Autodesk Fusion 360 part; units mm, degrees
(part 3 of 3)
sketch "Sketch8" plane through (0, 0, 4) normal (0, 0, 1) x (-1, 0, 0)
  arc A0 (-3.5192, 24.2905) -> (-4.2905, 23.5192) centre (0, 20) ccw
  arc A1 (-4.9606, 23.4245) -> (-4.2905, 23.5192) centre (-4.6771, 23.8363) ccw
  line L0 (-4.9606, 23.4245) -> (-6.1877, 24.2692)
  spline S0 degree 5 poles (-6.1877, 24.2692) (-6.1938, 24.2734) (-6.2062, 24.2817) (-6.2253, 24.2932) (-6.2514, 24.3073) (-6.2853, 24.3231) (-6.3199, 24.3375) (-6.355, 24.3512) (-6.3904, 24.3643) (-6.426, 24.3772) (-6.4618, 24.3897) (-6.4979, 24.4018) (-6.5343, 24.4132) (-6.571, 24.424) (-6.6082, 24.434) (-6.6457, 24.4434) (-6.6834, 24.4523) (-6.7214, 24.4607) (-6.7596, 24.4687) (-6.798, 24.4763) (-6.8365, 24.4835) (-6.8753, 24.4902) (-6.9143, 24.4965) (-6.9535, 24.5023) (-6.9928, 24.5077) (-7.0324, 24.5126) (-7.0722, 24.5171) (-7.1121, 24.5212) (-7.1522, 24.5249) (-7.1924, 24.5282) (-7.2328, 24.5311) (-7.2733, 24.5336) (-7.314, 24.5357) (-7.3548, 24.5374) (-7.3957, 24.5387) (-7.4368, 24.5396) (-7.478, 24.5402) (-7.5194, 24.5403) (-7.5608, 24.5401) (-7.6024, 24.5395) (-7.6441, 24.5386) (-7.6858, 24.5373) (-7.7277, 24.5356) (-7.7697, 24.5335) (-7.8118, 24.5311) (-7.854, 24.5283) (-7.8963, 24.5252) (-7.9386, 24.5217) (-7.9811, 24.5178) (-8.0236, 24.5136) (-8.0662, 24.509) (-8.1089, 24.5041) (-8.1517, 24.4988) (-8.1945, 24.4932) (-8.2374, 24.4872) (-8.2804, 24.4809) (-8.3234, 24.4742) (-8.3665, 24.4672) (-8.4097, 24.4598) (-8.4529, 24.4521) (-8.4961, 24.444) (-8.5394, 24.4357) (-8.5828, 24.4269) (-8.6261, 24.4179) (-8.6696, 24.4084) (-8.7131, 24.3987) (-8.7566, 24.3886) (-8.8001, 24.3782) (-8.8437, 24.3675) (-8.8873, 24.3564) (-8.9309, 24.345) (-8.9658, 24.3356) (-8.992, 24.3284) (-9.0095, 24.3235) (-9.0182, 24.321) knots 0 0 0 0 0 0 0.01428571 0.02857143 0.04285714 0.05714286 0.07142857 0.08571429 0.1 0.11428571 0.12857143 0.14285714 0.15714286 0.17142857 0.18571429 0.2 0.21428571 0.22857143 0.24285714 0.25714286 0.27142857 0.28571429 0.3 0.31428571 0.32857143 0.34285714 0.35714286 0.37142857 0.38571429 0.4 0.41428571 0.42857143 0.44285714 0.45714286 0.47142857 0.48571429 0.5 0.51428571 0.52857143 0.54285714 0.55714286 0.57142857 0.58571429 0.6 0.61428571 0.62857143 0.64285714 0.65714286 0.67142857 0.68571429 0.7 0.71428571 0.72857143 0.74285714 0.75714286 0.77142857 0.78571429 0.8 0.81428571 0.82857143 0.84285714 0.85714286 0.87142857 0.88571429 0.9 0.91428571 0.92857143 0.94285714 0.95714286 0.97142857 0.98571429 1 1 1 1 1 1
  arc A2 (-9.0182, 24.321) -> (-9.4323, 23.3214) centre (0, 20) ccw
  spline S1 degree 5 poles (-9.4323, 23.3214) (-9.4278, 23.3135) (-9.4189, 23.2977) (-9.4055, 23.2741) (-9.3874, 23.2427) (-9.3647, 23.2038) (-9.3417, 23.1652) (-9.3185, 23.1268) (-9.295, 23.0886) (-9.2714, 23.0507) (-9.2476, 23.0131) (-9.2235, 22.9757) (-9.1992, 22.9386) (-9.1748, 22.9018) (-9.1501, 22.8652) (-9.1252, 22.829) (-9.1001, 22.793) (-9.0748, 22.7573) (-9.0493, 22.7218) (-9.0236, 22.6867) (-8.9977, 22.6518) (-8.9716, 22.6173) (-8.9453, 22.583) (-8.9187, 22.549) (-8.892, 22.5153) (-8.8651, 22.482) (-8.8381, 22.4489) (-8.8108, 22.4162) (-8.7833, 22.3837) (-8.7556, 22.3516) (-8.7278, 22.3198) (-8.6997, 22.2883) (-8.6715, 22.2572) (-8.643, 22.2264) (-8.6144, 22.1959) (-8.5856, 22.1658) (-8.5567, 22.1359) (-8.5275, 22.1065) (-8.4981, 22.0774) (-8.4686, 22.0486) (-8.4389, 22.0202) (-8.409, 21.9922) (-8.379, 21.9646) (-8.3487, 21.9373) (-8.3183, 21.9104) (-8.2877, 21.8839) (-8.2569, 21.8578) (-8.226, 21.8321) (-8.1948, 21.8067) (-8.1636, 21.7818) (-8.1321, 21.7573) (-8.1005, 21.7332) (-8.0686, 21.7096) (-8.0366, 21.6865) (-8.0045, 21.6639) (-7.9721, 21.6417) (-7.9396, 21.6199) (-7.907, 21.5985) (-7.8742, 21.5776) (-7.8412, 21.5572) (-7.808, 21.5374) (-7.7746, 21.5182) (-7.741, 21.4998) (-7.7072, 21.4822) (-7.6732, 21.4652) (-7.639, 21.4487) (-7.6047, 21.4326) (-7.5704, 21.4169) (-7.5359, 21.4017) (-7.5013, 21.3875) (-7.4662, 21.3747) (-7.4377, 21.3661) (-7.416, 21.3609) (-7.4015, 21.3579) (-7.3941, 21.3565) knots -1 -1 -1 -1 -1 -1 -0.98571429 -0.97142857 -0.95714286 -0.94285714 -0.92857143 -0.91428571 -0.9 -0.88571429 -0.87142857 -0.85714286 -0.84285714 -0.82857143 -0.81428571 -0.8 -0.78571429 -0.77142857 -0.75714286 -0.74285714 -0.72857143 -0.71428571 -0.7 -0.68571429 -0.67142857 -0.65714286 -0.64285714 -0.62857143 -0.61428571 -0.6 -0.58571429 -0.57142857 -0.55714286 -0.54285714 -0.52857143 -0.51428571 -0.5 -0.48571429 -0.47142857 -0.45714286 -0.44285714 -0.42857143 -0.41428571 -0.4 -0.38571429 -0.37142857 -0.35714286 -0.34285714 -0.32857143 -0.31428571 -0.3 -0.28571429 -0.27142857 -0.25714286 -0.24285714 -0.22857143 -0.21428571 -0.2 -0.18571429 -0.17142857 -0.15714286 -0.14285714 -0.12857143 -0.11428571 -0.1 -0.08571429 -0.07142857 -0.05714286 -0.04285714 -0.02857143 -0.01428571 0 0 0 0 0 0
  line L1 (-7.3941, 21.3565) -> (-5.9292, 21.0862)
  arc A3 (-5.5223, 20.5454) -> (-5.9292, 21.0862) centre (-6.0199, 20.5945) ccw
  arc A4 (-5.5223, 20.5454) -> (-5.5223, 19.4546) centre (0, 20) ccw
  arc A5 (-5.9292, 18.9138) -> (-5.5223, 19.4546) centre (-6.0199, 19.4055) ccw
  line L2 (-5.9292, 18.9138) -> (-7.3941, 18.6435)
  spline S2 degree 5 poles (-7.3941, 18.6435) (-7.4015, 18.6421) (-7.416, 18.6391) (-7.4377, 18.6339) (-7.4662, 18.6253) (-7.5013, 18.6125) (-7.5359, 18.5983) (-7.5704, 18.5831) (-7.6047, 18.5674) (-7.639, 18.5513) (-7.6732, 18.5348) (-7.7072, 18.5178) (-7.741, 18.5002) (-7.7746, 18.4818) (-7.808, 18.4626) (-7.8412, 18.4428) (-7.8742, 18.4224) (-7.907, 18.4015) (-7.9396, 18.3801) (-7.9721, 18.3583) (-8.0045, 18.3361) (-8.0366, 18.3135) (-8.0686, 18.2904) (-8.1005, 18.2668) (-8.1321, 18.2427) (-8.1636, 18.2182) (-8.1948, 18.1933) (-8.226, 18.1679) (-8.2569, 18.1422) (-8.2877, 18.1161) (-8.3183, 18.0896) (-8.3487, 18.0627) (-8.379, 18.0354) (-8.409, 18.0078) (-8.4389, 17.9798) (-8.4686, 17.9514) (-8.4981, 17.9226) (-8.5275, 17.8935) (-8.5567, 17.8641) (-8.5856, 17.8343) (-8.6144, 17.8041) (-8.643, 17.7736) (-8.6715, 17.7428) (-8.6997, 17.7117) (-8.7278, 17.6802) (-8.7556, 17.6484) (-8.7833, 17.6163) (-8.8108, 17.5838) (-8.8381, 17.5511) (-8.8651, 17.518) (-8.892, 17.4847) (-8.9187, 17.451) (-8.9453, 17.417) (-8.9716, 17.3827) (-8.9977, 17.3482) (-9.0236, 17.3133) (-9.0493, 17.2782) (-9.0748, 17.2427) (-9.1001, 17.207) (-9.1252, 17.171) (-9.1501, 17.1348) (-9.1748, 17.0982) (-9.1992, 17.0614) (-9.2235, 17.0243) (-9.2476, 16.9869) (-9.2714, 16.9493) (-9.295, 16.9114) (-9.3185, 16.8733) (-9.3417, 16.8348) (-9.3647, 16.7962) (-9.3874, 16.7573) (-9.4055, 16.7259) (-9.4189, 16.7023) (-9.4278, 16.6865) (-9.4323, 16.6786) knots 0 0 0 0 0 0 0.01428571 0.02857143 0.04285714 0.05714286 0.07142857 0.08571429 0.1 0.11428571 0.12857143 0.14285714 0.15714286 0.17142857 0.18571429 0.2 0.21428571 0.22857143 0.24285714 0.25714286 0.27142857 0.28571429 0.3 0.31428571 0.32857143 0.34285714 0.35714286 0.37142857 0.38571429 0.4 0.41428571 0.42857143 0.44285714 0.45714286 0.47142857 0.48571429 0.5 0.51428571 0.52857143 0.54285714 0.55714286 0.57142857 0.58571429 0.6 0.61428571 0.62857143 0.64285714 0.65714286 0.67142857 0.68571429 0.7 0.71428571 0.72857143 0.74285714 0.75714286 0.77142857 0.78571429 0.8 0.81428571 0.82857143 0.84285714 0.85714286 0.87142857 0.88571429 0.9 0.91428571 0.92857143 0.94285714 0.95714286 0.97142857 0.98571429 1 1 1 1 1 1
  arc A6 (-9.4323, 16.6786) -> (-9.0182, 15.679) centre (0, 20) ccw
  spline S3 degree 5 poles (-9.0182, 15.679) (-9.0095, 15.6765) (-8.992, 15.6716) (-8.9658, 15.6644) (-8.9309, 15.655) (-8.8873, 15.6436) (-8.8437, 15.6325) (-8.8001, 15.6218) (-8.7566, 15.6114) (-8.7131, 15.6013) (-8.6696, 15.5916) (-8.6261, 15.5821) (-8.5828, 15.5731) (-8.5394, 15.5643) (-8.4961, 15.556) (-8.4529, 15.5479) (-8.4097, 15.5402) (-8.3665, 15.5328) (-8.3234, 15.5258) (-8.2804, 15.5191) (-8.2374, 15.5128) (-8.1945, 15.5068) (-8.1517, 15.5012) (-8.1089, 15.4959) (-8.0662, 15.491) (-8.0236, 15.4864) (-7.9811, 15.4822) (-7.9386, 15.4783) (-7.8963, 15.4748) (-7.854, 15.4717) (-7.8118, 15.4689) (-7.7697, 15.4665) (-7.7277, 15.4644) (-7.6858, 15.4627) (-7.6441, 15.4614) (-7.6024, 15.4605) (-7.5608, 15.4599) (-7.5194, 15.4597) (-7.478, 15.4598) (-7.4368, 15.4604) (-7.3957, 15.4613) (-7.3548, 15.4626) (-7.314, 15.4643) (-7.2733, 15.4664) (-7.2328, 15.4689) (-7.1924, 15.4718) (-7.1522, 15.4751) (-7.1121, 15.4788) (-7.0722, 15.4829) (-7.0324, 15.4874) (-6.9928, 15.4923) (-6.9535, 15.4977) (-6.9143, 15.5035) (-6.8753, 15.5098) (-6.8365, 15.5165) (-6.798, 15.5237) (-6.7596, 15.5313) (-6.7214, 15.5393) (-6.6834, 15.5477) (-6.6457, 15.5566) (-6.6082, 15.566) (-6.571, 15.576) (-6.5343, 15.5868) (-6.4979, 15.5982) (-6.4618, 15.6103) (-6.426, 15.6228) (-6.3904, 15.6357) (-6.355, 15.6488) (-6.3199, 15.6625) (-6.2853, 15.6769) (-6.2514, 15.6927) (-6.2253, 15.7068) (-6.2062, 15.7183) (-6.1938, 15.7266) (-6.1877, 15.7308) knots -1 -1 -1 -1 -1 -1 -0.98571429 -0.97142857 -0.95714286 -0.94285714 -0.92857143 -0.91428571 -0.9 -0.88571429 -0.87142857 -0.85714286 -0.84285714 -0.82857143 -0.81428571 -0.8 -0.78571429 -0.77142857 -0.75714286 -0.74285714 -0.72857143 -0.71428571 -0.7 -0.68571429 -0.67142857 -0.65714286 -0.64285714 -0.62857143 -0.61428571 -0.6 -0.58571429 -0.57142857 -0.55714286 -0.54285714 -0.52857143 -0.51428571 -0.5 -0.48571429 -0.47142857 -0.45714286 -0.44285714 -0.42857143 -0.41428571 -0.4 -0.38571429 -0.37142857 -0.35714286 -0.34285714 -0.32857143 -0.31428571 -0.3 -0.28571429 -0.27142857 -0.25714286 -0.24285714 -0.22857143 -0.21428571 -0.2 -0.18571429 -0.17142857 -0.15714286 -0.14285714 -0.12857143 -0.11428571 -0.1 -0.08571429 -0.07142857 -0.05714286 -0.04285714 -0.02857143 -0.01428571 0 0 0 0 0 0
  line L3 (-6.1877, 15.7308) -> (-4.9606, 16.5755)
  arc A7 (-4.2905, 16.4808) -> (-4.9606, 16.5755) centre (-4.6771, 16.1637) ccw
  arc A8 (-4.2905, 16.4808) -> (-3.5192, 15.7095) centre (0, 20) ccw
  arc A9 (-3.4245, 15.0394) -> (-3.5192, 15.7095) centre (-3.8363, 15.3229) ccw
  line L4 (-3.4245, 15.0394) -> (-4.2692, 13.8123)
  spline S4 degree 5 poles (-4.2692, 13.8123) (-4.2734, 13.8062) (-4.2817, 13.7938) (-4.2932, 13.7747) (-4.3073, 13.7486) (-4.3231, 13.7147) (-4.3375, 13.6801) (-4.3512, 13.645) (-4.3643, 13.6096) (-4.3772, 13.574) (-4.3897, 13.5382) (-4.4018, 13.5021) (-4.4132, 13.4657) (-4.424, 13.429) (-4.434, 13.3918) (-4.4434, 13.3543) (-4.4523, 13.3166) (-4.4607, 13.2786) (-4.4687, 13.2404) (-4.4763, 13.202) (-4.4835, 13.1635) (-4.4902, 13.1247) (-4.4965, 13.0857) (-4.5023, 13.0465) (-4.5077, 13.0072) (-4.5126, 12.9676) (-4.5171, 12.9278) (-4.5212, 12.8879) (-4.5249, 12.8478) (-4.5282, 12.8076) (-4.5311, 12.7672) (-4.5336, 12.7267) (-4.5357, 12.686) (-4.5374, 12.6452) (-4.5387, 12.6043) (-4.5396, 12.5632) (-4.5402, 12.522) (-4.5403, 12.4806) (-4.5401, 12.4392) (-4.5395, 12.3976) (-4.5386, 12.3559) (-4.5373, 12.3142) (-4.5356, 12.2723) (-4.5335, 12.2303) (-4.5311, 12.1882) (-4.5283, 12.146) (-4.5252, 12.1037) (-4.5217, 12.0614) (-4.5178, 12.0189) (-4.5136, 11.9764) (-4.509, 11.9338) (-4.5041, 11.8911) (-4.4988, 11.8483) (-4.4932, 11.8055) (-4.4872, 11.7626) (-4.4809, 11.7196) (-4.4742, 11.6766) (-4.4672, 11.6335) (-4.4598, 11.5903) (-4.4521, 11.5471) (-4.444, 11.5039) (-4.4357, 11.4606) (-4.4269, 11.4172) (-4.4179, 11.3739) (-4.4084, 11.3304) (-4.3987, 11.2869) (-4.3886, 11.2434) (-4.3782, 11.1999) (-4.3675, 11.1563) (-4.3564, 11.1127) (-4.345, 11.0691) (-4.3356, 11.0342) (-4.3284, 11.008) (-4.3235, 10.9905) (-4.321, 10.9818) knots 0 0 0 0 0 0 0.01428571 0.02857143 0.04285714 0.05714286 0.07142857 0.08571429 0.1 0.11428571 0.12857143 0.14285714 0.15714286 0.17142857 0.18571429 0.2 0.21428571 0.22857143 0.24285714 0.25714286 0.27142857 0.28571429 0.3 0.31428571 0.32857143 0.34285714 0.35714286 0.37142857 0.38571429 0.4 0.41428571 0.42857143 0.44285714 0.45714286 0.47142857 0.48571429 0.5 0.51428571 0.52857143 0.54285714 0.55714286 0.57142857 0.58571429 0.6 0.61428571 0.62857143 0.64285714 0.65714286 0.67142857 0.68571429 0.7 0.71428571 0.72857143 0.74285714 0.75714286 0.77142857 0.78571429 0.8 0.81428571 0.82857143 0.84285714 0.85714286 0.87142857 0.88571429 0.9 0.91428571 0.92857143 0.94285714 0.95714286 0.97142857 0.98571429 1 1 1 1 1 1
  arc A10 (-4.321, 10.9818) -> (-3.3214, 10.5677) centre (0, 20) ccw
  spline S5 degree 5 poles (-3.3214, 10.5677) (-3.3135, 10.5722) (-3.2977, 10.5811) (-3.2741, 10.5945) (-3.2427, 10.6126) (-3.2038, 10.6353) (-3.1652, 10.6583) (-3.1267, 10.6815) (-3.0886, 10.705) (-3.0507, 10.7286) (-3.0131, 10.7524) (-2.9757, 10.7765) (-2.9386, 10.8008) (-2.9018, 10.8252) (-2.8652, 10.8499) (-2.829, 10.8748) (-2.793, 10.8999) (-2.7573, 10.9252) (-2.7218, 10.9507) (-2.6867, 10.9764) (-2.6518, 11.0023) (-2.6173, 11.0284) (-2.583, 11.0547) (-2.549, 11.0813) (-2.5153, 11.108) (-2.482, 11.1349) (-2.4489, 11.1619) (-2.4162, 11.1892) (-2.3837, 11.2167) (-2.3516, 11.2444) (-2.3198, 11.2722) (-2.2883, 11.3003) (-2.2572, 11.3285) (-2.2264, 11.357) (-2.1959, 11.3856) (-2.1657, 11.4144) (-2.1359, 11.4433) (-2.1065, 11.4725) (-2.0774, 11.5019) (-2.0486, 11.5314) (-2.0202, 11.5611) (-1.9922, 11.591) (-1.9646, 11.621) (-1.9373, 11.6513) (-1.9104, 11.6817) (-1.8839, 11.7123) (-1.8578, 11.7431) (-1.8321, 11.774) (-1.8067, 11.8052) (-1.7818, 11.8364) (-1.7573, 11.8679) (-1.7332, 11.8995) (-1.7096, 11.9314) (-1.6865, 11.9634) (-1.6639, 11.9955) (-1.6417, 12.0279) (-1.6199, 12.0604) (-1.5985, 12.093) (-1.5776, 12.1258) (-1.5572, 12.1588) (-1.5374, 12.192) (-1.5182, 12.2254) (-1.4998, 12.259) (-1.4822, 12.2928) (-1.4652, 12.3268) (-1.4487, 12.361) (-1.4326, 12.3953) (-1.4169, 12.4296) (-1.4017, 12.4641) (-1.3875, 12.4987) (-1.3747, 12.5338) (-1.3661, 12.5623) (-1.3609, 12.584) (-1.3579, 12.5985) (-1.3565, 12.6059) knots -1 -1 -1 -1 -1 -1 -0.98571429 -0.97142857 -0.95714286 -0.94285714 -0.92857143 -0.91428571 -0.9 -0.88571429 -0.87142857 -0.85714286 -0.84285714 -0.82857143 -0.81428571 -0.8 -0.78571429 -0.77142857 -0.75714286 -0.74285714 -0.72857143 -0.71428571 -0.7 -0.68571429 -0.67142857 -0.65714286 -0.64285714 -0.62857143 -0.61428571 -0.6 -0.58571429 -0.57142857 -0.55714286 -0.54285714 -0.52857143 -0.51428571 -0.5 -0.48571429 -0.47142857 -0.45714286 -0.44285714 -0.42857143 -0.41428571 -0.4 -0.38571429 -0.37142857 -0.35714286 -0.34285714 -0.32857143 -0.31428571 -0.3 -0.28571429 -0.27142857 -0.25714286 -0.24285714 -0.22857143 -0.21428571 -0.2 -0.18571429 -0.17142857 -0.15714286 -0.14285714 -0.12857143 -0.11428571 -0.1 -0.08571429 -0.07142857 -0.05714286 -0.04285714 -0.02857143 -0.01428571 0 0 0 0 0 0
  line L5 (-1.3565, 12.6059) -> (-1.0862, 14.0708)
  arc A11 (-0.5454, 14.4777) -> (-1.0862, 14.0708) centre (-0.5945, 13.9801) ccw
  arc A12 (-0.5454, 14.4777) -> (0.5454, 14.4777) centre (0, 20) ccw
  arc A13 (1.0862, 14.0708) -> (0.5454, 14.4777) centre (0.5945, 13.9801) ccw
  line L6 (1.0862, 14.0708) -> (1.3565, 12.6059)
  spline S6 degree 5 poles (1.3565, 12.6059) (1.3579, 12.5985) (1.3609, 12.584) (1.3661, 12.5623) (1.3747, 12.5338) (1.3875, 12.4987) (1.4017, 12.4641) (1.4169, 12.4296) (1.4326, 12.3953) (1.4487, 12.361) (1.4652, 12.3268) (1.4822, 12.2928) (1.4998, 12.259) (1.5182, 12.2254) (1.5374, 12.192) (1.5572, 12.1588) (1.5776, 12.1258) (1.5985, 12.093) (1.6199, 12.0604) (1.6417, 12.0279) (1.6639, 11.9955) (1.6865, 11.9634) (1.7096, 11.9314) (1.7332, 11.8995) (1.7573, 11.8679) (1.7818, 11.8364) (1.8067, 11.8052) (1.8321, 11.774) (1.8578, 11.7431) (1.8839, 11.7123) (1.9104, 11.6817) (1.9373, 11.6513) (1.9646, 11.621) (1.9922, 11.591) (2.0202, 11.5611) (2.0486, 11.5314) (2.0774, 11.5019) (2.1065, 11.4725) (2.1359, 11.4433) (2.1657, 11.4144) (2.1959, 11.3856) (2.2264, 11.357) (2.2572, 11.3285) (2.2883, 11.3003) (2.3198, 11.2722) (2.3516, 11.2444) (2.3837, 11.2167) (2.4162, 11.1892) (2.4489, 11.1619) (2.482, 11.1349) (2.5153, 11.108) (2.549, 11.0813) (2.583, 11.0547) (2.6173, 11.0284) (2.6518, 11.0023) (2.6867, 10.9764) (2.7218, 10.9507) (2.7573, 10.9252) (2.793, 10.8999) (2.829, 10.8748) (2.8652, 10.8499) (2.9018, 10.8252) (2.9386, 10.8008) (2.9757, 10.7765) (3.0131, 10.7524) (3.0507, 10.7286) (3.0886, 10.705) (3.1267, 10.6815) (3.1652, 10.6583) (3.2038, 10.6353) (3.2427, 10.6126) (3.2741, 10.5945) (3.2977, 10.5811) (3.3135, 10.5722) (3.3214, 10.5677) knots 0 0 0 0 0 0 0.01428571 0.02857143 0.04285714 0.05714286 0.07142857 0.08571429 0.1 0.11428571 0.12857143 0.14285714 0.15714286 0.17142857 0.18571429 0.2 0.21428571 0.22857143 0.24285714 0.25714286 0.27142857 0.28571429 0.3 0.31428571 0.32857143 0.34285714 0.35714286 0.37142857 0.38571429 0.4 0.41428571 0.42857143 0.44285714 0.45714286 0.47142857 0.48571429 0.5 0.51428571 0.52857143 0.54285714 0.55714286 0.57142857 0.58571429 0.6 0.61428571 0.62857143 0.64285714 0.65714286 0.67142857 0.68571429 0.7 0.71428571 0.72857143 0.74285714 0.75714286 0.77142857 0.78571429 0.8 0.81428571 0.82857143 0.84285714 0.85714286 0.87142857 0.88571429 0.9 0.91428571 0.92857143 0.94285714 0.95714286 0.97142857 0.98571429 1 1 1 1 1 1
  arc A14 (3.3214, 10.5677) -> (4.321, 10.9818) centre (0, 20) ccw
  spline S7 degree 5 poles (4.321, 10.9818) (4.3235, 10.9905) (4.3284, 11.008) (4.3356, 11.0342) (4.345, 11.0691) (4.3564, 11.1127) (4.3675, 11.1563) (4.3782, 11.1999) (4.3886, 11.2434) (4.3987, 11.2869) (4.4084, 11.3304) (4.4179, 11.3739) (4.4269, 11.4172) (4.4357, 11.4606) (4.444, 11.5039) (4.4521, 11.5471) (4.4598, 11.5903) (4.4672, 11.6335) (4.4742, 11.6766) (4.4809, 11.7196) (4.4872, 11.7626) (4.4932, 11.8055) (4.4988, 11.8483) (4.5041, 11.8911) (4.509, 11.9338) (4.5136, 11.9764) (4.5178, 12.0189) (4.5217, 12.0614) (4.5252, 12.1037) (4.5283, 12.146) (4.5311, 12.1882) (4.5335, 12.2303) (4.5356, 12.2723) (4.5373, 12.3142) (4.5386, 12.3559) (4.5395, 12.3976) (4.5401, 12.4392) (4.5403, 12.4806) (4.5402, 12.522) (4.5396, 12.5632) (4.5387, 12.6043) (4.5374, 12.6452) (4.5357, 12.686) (4.5336, 12.7267) (4.5311, 12.7672) (4.5282, 12.8076) (4.5249, 12.8478) (4.5212, 12.8879) (4.5171, 12.9278) (4.5126, 12.9676) (4.5077, 13.0072) (4.5023, 13.0465) (4.4965, 13.0857) (4.4902, 13.1247) (4.4835, 13.1635) (4.4763, 13.202) (4.4687, 13.2404) (4.4607, 13.2786) (4.4523, 13.3166) (4.4434, 13.3543) (4.434, 13.3918) (4.424, 13.429) (4.4132, 13.4657) (4.4018, 13.5021) (4.3897, 13.5382) (4.3772, 13.574) (4.3643, 13.6096) (4.3512, 13.645) (4.3375, 13.6801) (4.3231, 13.7147) (4.3073, 13.7486) (4.2932, 13.7747) (4.2817, 13.7938) (4.2734, 13.8062) (4.2692, 13.8123) knots -1 -1 -1 -1 -1 -1 -0.98571429 -0.97142857 -0.95714286 -0.94285714 -0.92857143 -0.91428571 -0.9 -0.88571429 -0.87142857 -0.85714286 -0.84285714 -0.82857143 -0.81428571 -0.8 -0.78571429 -0.77142857 -0.75714286 -0.74285714 -0.72857143 -0.71428571 -0.7 -0.68571429 -0.67142857 -0.65714286 -0.64285714 -0.62857143 -0.61428571 -0.6 -0.58571429 -0.57142857 -0.55714286 -0.54285714 -0.52857143 -0.51428571 -0.5 -0.48571429 -0.47142857 -0.45714286 -0.44285714 -0.42857143 -0.41428571 -0.4 -0.38571429 -0.37142857 -0.35714286 -0.34285714 -0.32857143 -0.31428571 -0.3 -0.28571429 -0.27142857 -0.25714286 -0.24285714 -0.22857143 -0.21428571 -0.2 -0.18571429 -0.17142857 -0.15714286 -0.14285714 -0.12857143 -0.11428571 -0.1 -0.08571429 -0.07142857 -0.05714286 -0.04285714 -0.02857143 -0.01428571 0 0 0 0 0 0
  line L7 (4.2692, 13.8123) -> (3.4245, 15.0394)
  arc A15 (3.5192, 15.7095) -> (3.4245, 15.0394) centre (3.8363, 15.3229) ccw
  arc A16 (3.5192, 15.7095) -> (4.2905, 16.4808) centre (0, 20) ccw
  arc A17 (4.9606, 16.5755) -> (4.2905, 16.4808) centre (4.6771, 16.1637) ccw
  line L8 (4.9606, 16.5755) -> (6.1877, 15.7308)
  spline S8 degree 5 poles (6.1877, 15.7308) (6.1938, 15.7266) (6.2062, 15.7183) (6.2253, 15.7068) (6.2514, 15.6927) (6.2853, 15.6769) (6.3199, 15.6625) (6.355, 15.6488) (6.3904, 15.6357) (6.426, 15.6228) (6.4618, 15.6103) (6.4979, 15.5982) (6.5343, 15.5868) (6.571, 15.576) (6.6082, 15.566) (6.6457, 15.5566) (6.6834, 15.5477) (6.7214, 15.5393) (6.7596, 15.5313) (6.798, 15.5237) (6.8365, 15.5165) (6.8753, 15.5098) (6.9143, 15.5035) (6.9535, 15.4977) (6.9928, 15.4923) (7.0324, 15.4874) (7.0722, 15.4829) (7.1121, 15.4788) (7.1522, 15.4751) (7.1924, 15.4718) (7.2328, 15.4689) (7.2733, 15.4664) (7.314, 15.4643) (7.3548, 15.4626) (7.3957, 15.4613) (7.4368, 15.4604) (7.478, 15.4598) (7.5194, 15.4597) (7.5608, 15.4599) (7.6024, 15.4605) (7.6441, 15.4614) (7.6858, 15.4627) (7.7277, 15.4644) (7.7697, 15.4665) (7.8118, 15.4689) (7.854, 15.4717) (7.8963, 15.4748) (7.9386, 15.4783) (7.9811, 15.4822) (8.0236, 15.4864) (8.0662, 15.491) (8.1089, 15.4959) (8.1517, 15.5012) (8.1945, 15.5068) (8.2374, 15.5128) (8.2804, 15.5191) (8.3234, 15.5258) (8.3665, 15.5328) (8.4097, 15.5402) (8.4529, 15.5479) (8.4961, 15.556) (8.5394, 15.5643) (8.5828, 15.5731) (8.6261, 15.5821) (8.6696, 15.5916) (8.7131, 15.6013) (8.7566, 15.6114) (8.8001, 15.6218) (8.8437, 15.6325) (8.8873, 15.6436) (8.9309, 15.655) (8.9658, 15.6644) (8.992, 15.6716) (9.0095, 15.6765) (9.0182, 15.679) knots 0 0 0 0 0 0 0.01428571 0.02857143 0.04285714 0.05714286 0.07142857 0.08571429 0.1 0.11428571 0.12857143 0.14285714 0.15714286 0.17142857 0.18571429 0.2 0.21428571 0.22857143 0.24285714 0.25714286 0.27142857 0.28571429 0.3 0.31428571 0.32857143 0.34285714 0.35714286 0.37142857 0.38571429 0.4 0.41428571 0.42857143 0.44285714 0.45714286 0.47142857 0.48571429 0.5 0.51428571 0.52857143 0.54285714 0.55714286 0.57142857 0.58571429 0.6 0.61428571 0.62857143 0.64285714 0.65714286 0.67142857 0.68571429 0.7 0.71428571 0.72857143 0.74285714 0.75714286 0.77142857 0.78571429 0.8 0.81428571 0.82857143 0.84285714 0.85714286 0.87142857 0.88571429 0.9 0.91428571 0.92857143 0.94285714 0.95714286 0.97142857 0.98571429 1 1 1 1 1 1
  arc A18 (9.0182, 15.679) -> (9.4323, 16.6786) centre (0, 20) ccw
  spline S9 degree 5 poles (9.4323, 16.6786) (9.4278, 16.6865) (9.4189, 16.7023) (9.4055, 16.7259) (9.3874, 16.7573) (9.3647, 16.7962) (9.3417, 16.8348) (9.3185, 16.8733) (9.295, 16.9114) (9.2714, 16.9493) (9.2476, 16.9869) (9.2235, 17.0243) (9.1992, 17.0614) (9.1748, 17.0982) (9.1501, 17.1348) (9.1252, 17.171) (9.1001, 17.207) (9.0748, 17.2427) (9.0493, 17.2782) (9.0236, 17.3133) (8.9977, 17.3482) (8.9716, 17.3827) (8.9453, 17.417) (8.9187, 17.451) (8.892, 17.4847) (8.8651, 17.518) (8.8381, 17.5511) (8.8108, 17.5838) (8.7833, 17.6163) (8.7556, 17.6484) (8.7278, 17.6802) (8.6997, 17.7117) (8.6715, 17.7428) (8.643, 17.7736) (8.6144, 17.8041) (8.5856, 17.8343) (8.5567, 17.8641) (8.5275, 17.8935) (8.4981, 17.9226) (8.4686, 17.9514) (8.4389, 17.9798) (8.409, 18.0078) (8.379, 18.0354) (8.3487, 18.0627) (8.3183, 18.0896) (8.2877, 18.1161) (8.2569, 18.1422) (8.226, 18.1679) (8.1948, 18.1933) (8.1636, 18.2182) (8.1321, 18.2427) (8.1005, 18.2668) (8.0686, 18.2904) (8.0366, 18.3135) (8.0045, 18.3361) (7.9721, 18.3583) (7.9396, 18.3801) (7.907, 18.4015) (7.8742, 18.4224) (7.8412, 18.4428) (7.808, 18.4626) (7.7746, 18.4818) (7.741, 18.5002) (7.7072, 18.5178) (7.6732, 18.5348) (7.639, 18.5513) (7.6047, 18.5674) (7.5704, 18.5831) (7.5359, 18.5983) (7.5013, 18.6125) (7.4662, 18.6253) (7.4377, 18.6339) (7.416, 18.6391) (7.4015, 18.6421) (7.3941, 18.6435) knots -1 -1 -1 -1 -1 -1 -0.98571429 -0.97142857 -0.95714286 -0.94285714 -0.92857143 -0.91428571 -0.9 -0.88571429 -0.87142857 -0.85714286 -0.84285714 -0.82857143 -0.81428571 -0.8 -0.78571429 -0.77142857 -0.75714286 -0.74285714 -0.72857143 -0.71428571 -0.7 -0.68571429 -0.67142857 -0.65714286 -0.64285714 -0.62857143 -0.61428571 -0.6 -0.58571429 -0.57142857 -0.55714286 -0.54285714 -0.52857143 -0.51428571 -0.5 -0.48571429 -0.47142857 -0.45714286 -0.44285714 -0.42857143 -0.41428571 -0.4 -0.38571429 -0.37142857 -0.35714286 -0.34285714 -0.32857143 -0.31428571 -0.3 -0.28571429 -0.27142857 -0.25714286 -0.24285714 -0.22857143 -0.21428571 -0.2 -0.18571429 -0.17142857 -0.15714286 -0.14285714 -0.12857143 -0.11428571 -0.1 -0.08571429 -0.07142857 -0.05714286 -0.04285714 -0.02857143 -0.01428571 0 0 0 0 0 0
  line L9 (7.3941, 18.6435) -> (5.9292, 18.9138)
  arc A19 (5.5223, 19.4546) -> (5.9292, 18.9138) centre (6.0199, 19.4055) ccw
  arc A20 (5.5223, 19.4546) -> (5.5223, 20.5454) centre (0, 20) ccw
  arc A21 (5.9292, 21.0862) -> (5.5223, 20.5454) centre (6.0199, 20.5945) ccw
  line L10 (5.9292, 21.0862) -> (7.3941, 21.3565)
  spline S10 degree 5 poles (7.3941, 21.3565) (7.4015, 21.3579) (7.416, 21.3609) (7.4377, 21.3661) (7.4662, 21.3747) (7.5013, 21.3875) (7.5359, 21.4017) (7.5704, 21.4169) (7.6047, 21.4326) (7.639, 21.4487) (7.6732, 21.4652) (7.7072, 21.4822) (7.741, 21.4998) (7.7746, 21.5182) (7.808, 21.5374) (7.8412, 21.5572) (7.8742, 21.5776) (7.907, 21.5985) (7.9396, 21.6199) (7.9721, 21.6417) (8.0045, 21.6639) (8.0366, 21.6865) (8.0686, 21.7096) (8.1005, 21.7332) (8.1321, 21.7573) (8.1636, 21.7818) (8.1948, 21.8067) (8.226, 21.8321) (8.2569, 21.8578) (8.2877, 21.8839) (8.3183, 21.9104) (8.3487, 21.9373) (8.379, 21.9646) (8.409, 21.9922) (8.4389, 22.0202) (8.4686, 22.0486) (8.4981, 22.0774) (8.5275, 22.1065) (8.5567, 22.1359) (8.5856, 22.1658) (8.6144, 22.1959) (8.643, 22.2264) (8.6715, 22.2572) (8.6997, 22.2883) (8.7278, 22.3198) (8.7556, 22.3516) (8.7833, 22.3837) (8.8108, 22.4162) (8.8381, 22.4489) (8.8651, 22.482) (8.892, 22.5153) (8.9187, 22.549) (8.9453, 22.583) (8.9716, 22.6173) (8.9977, 22.6518) (9.0236, 22.6867) (9.0493, 22.7218) (9.0748, 22.7573) (9.1001, 22.793) (9.1252, 22.829) (9.1501, 22.8652) (9.1748, 22.9018) (9.1992, 22.9386) (9.2235, 22.9757) (9.2476, 23.0131) (9.2714, 23.0507) (9.295, 23.0886) (9.3185, 23.1268) (9.3417, 23.1652) (9.3647, 23.2038) (9.3874, 23.2427) (9.4055, 23.2741) (9.4189, 23.2977) (9.4278, 23.3135) (9.4323, 23.3214) knots 0 0 0 0 0 0 0.01428571 0.02857143 0.04285714 0.05714286 0.07142857 0.08571429 0.1 0.11428571 0.12857143 0.14285714 0.15714286 0.17142857 0.18571429 0.2 0.21428571 0.22857143 0.24285714 0.25714286 0.27142857 0.28571429 0.3 0.31428571 0.32857143 0.34285714 0.35714286 0.37142857 0.38571429 0.4 0.41428571 0.42857143 0.44285714 0.45714286 0.47142857 0.48571429 0.5 0.51428571 0.52857143 0.54285714 0.55714286 0.57142857 0.58571429 0.6 0.61428571 0.62857143 0.64285714 0.65714286 0.67142857 0.68571429 0.7 0.71428571 0.72857143 0.74285714 0.75714286 0.77142857 0.78571429 0.8 0.81428571 0.82857143 0.84285714 0.85714286 0.87142857 0.88571429 0.9 0.91428571 0.92857143 0.94285714 0.95714286 0.97142857 0.98571429 1 1 1 1 1 1
  arc A22 (9.4323, 23.3214) -> (9.0182, 24.321) centre (0, 20) ccw
  spline S11 degree 5 poles (9.0182, 24.321) (9.0095, 24.3235) (8.992, 24.3284) (8.9658, 24.3356) (8.9309, 24.345) (8.8873, 24.3564) (8.8437, 24.3675) (8.8001, 24.3782) (8.7566, 24.3886) (8.7131, 24.3987) (8.6696, 24.4084) (8.6261, 24.4179) (8.5828, 24.4269) (8.5394, 24.4357) (8.4961, 24.444) (8.4529, 24.4521) (8.4097, 24.4598) (8.3665, 24.4672) (8.3234, 24.4742) (8.2804, 24.4809) (8.2374, 24.4872) (8.1945, 24.4932) (8.1517, 24.4988) (8.1089, 24.5041) (8.0662, 24.509) (8.0236, 24.5136) (7.9811, 24.5178) (7.9386, 24.5217) (7.8963, 24.5252) (7.854, 24.5283) (7.8118, 24.5311) (7.7697, 24.5335) (7.7277, 24.5356) (7.6858, 24.5373) (7.6441, 24.5386) (7.6024, 24.5395) (7.5608, 24.5401) (7.5194, 24.5403) (7.478, 24.5402) (7.4368, 24.5396) (7.3957, 24.5387) (7.3548, 24.5374) (7.314, 24.5357) (7.2733, 24.5336) (7.2328, 24.5311) (7.1924, 24.5282) (7.1522, 24.5249) (7.1121, 24.5212) (7.0722, 24.5171) (7.0324, 24.5126) (6.9928, 24.5077) (6.9535, 24.5023) (6.9143, 24.4965) (6.8753, 24.4902) (6.8365, 24.4835) (6.798, 24.4763) (6.7596, 24.4687) (6.7214, 24.4607) (6.6834, 24.4523) (6.6457, 24.4434) (6.6082, 24.434) (6.571, 24.424) (6.5343, 24.4132) (6.4979, 24.4018) (6.4618, 24.3897) (6.426, 24.3772) (6.3904, 24.3643) (6.355, 24.3512) (6.3199, 24.3375) (6.2853, 24.3231) (6.2514, 24.3073) (6.2253, 24.2932) (6.2062, 24.2817) (6.1938, 24.2734) (6.1877, 24.2692) knots -1 -1 -1 -1 -1 -1 -0.98571429 -0.97142857 -0.95714286 -0.94285714 -0.92857143 -0.91428571 -0.9 -0.88571429 -0.87142857 -0.85714286 -0.84285714 -0.82857143 -0.81428571 -0.8 -0.78571429 -0.77142857 -0.75714286 -0.74285714 -0.72857143 -0.71428571 -0.7 -0.68571429 -0.67142857 -0.65714286 -0.64285714 -0.62857143 -0.61428571 -0.6 -0.58571429 -0.57142857 -0.55714286 -0.54285714 -0.52857143 -0.51428571 -0.5 -0.48571429 -0.47142857 -0.45714286 -0.44285714 -0.42857143 -0.41428571 -0.4 -0.38571429 -0.37142857 -0.35714286 -0.34285714 -0.32857143 -0.31428571 -0.3 -0.28571429 -0.27142857 -0.25714286 -0.24285714 -0.22857143 -0.21428571 -0.2 -0.18571429 -0.17142857 -0.15714286 -0.14285714 -0.12857143 -0.11428571 -0.1 -0.08571429 -0.07142857 -0.05714286 -0.04285714 -0.02857143 -0.01428571 0 0 0 0 0 0
  line L11 (6.1877, 24.2692) -> (4.9606, 23.4245)
  arc A23 (4.2905, 23.5192) -> (4.9606, 23.4245) centre (4.6771, 23.8363) ccw
  arc A24 (4.2905, 23.5192) -> (3.5192, 24.2905) centre (0, 20) ccw
  arc A25 (3.4245, 24.9606) -> (3.5192, 24.2905) centre (3.8363, 24.6771) ccw
  line L12 (3.4245, 24.9606) -> (4.2692, 26.1877)
  spline S12 degree 5 poles (4.2692, 26.1877) (4.2734, 26.1938) (4.2817, 26.2062) (4.2932, 26.2253) (4.3073, 26.2514) (4.3231, 26.2853) (4.3375, 26.3199) (4.3512, 26.355) (4.3643, 26.3904) (4.3772, 26.426) (4.3897, 26.4618) (4.4018, 26.4979) (4.4132, 26.5343) (4.424, 26.5711) (4.434, 26.6082) (4.4434, 26.6457) (4.4523, 26.6834) (4.4607, 26.7214) (4.4687, 26.7596) (4.4763, 26.798) (4.4835, 26.8365) (4.4902, 26.8753) (4.4965, 26.9143) (4.5023, 26.9535) (4.5077, 26.9928) (4.5126, 27.0324) (4.5171, 27.0722) (4.5212, 27.1121) (4.5249, 27.1522) (4.5282, 27.1924) (4.5311, 27.2328) (4.5336, 27.2733) (4.5357, 27.314) (4.5374, 27.3548) (4.5387, 27.3957) (4.5396, 27.4368) (4.5402, 27.478) (4.5403, 27.5194) (4.5401, 27.5608) (4.5395, 27.6024) (4.5386, 27.6441) (4.5373, 27.6858) (4.5356, 27.7277) (4.5335, 27.7697) (4.5311, 27.8118) (4.5283, 27.854) (4.5252, 27.8963) (4.5217, 27.9386) (4.5178, 27.9811) (4.5136, 28.0236) (4.509, 28.0662) (4.5041, 28.1089) (4.4988, 28.1517) (4.4932, 28.1945) (4.4872, 28.2374) (4.4809, 28.2804) (4.4742, 28.3234) (4.4672, 28.3665) (4.4598, 28.4097) (4.4521, 28.4529) (4.444, 28.4961) (4.4357, 28.5394) (4.4269, 28.5828) (4.4179, 28.6261) (4.4084, 28.6696) (4.3987, 28.7131) (4.3886, 28.7566) (4.3782, 28.8001) (4.3675, 28.8437) (4.3564, 28.8873) (4.345, 28.9309) (4.3356, 28.9658) (4.3284, 28.992) (4.3235, 29.0095) (4.321, 29.0182) knots 0 0 0 0 0 0 0.01428571 0.02857143 0.04285714 0.05714286 0.07142857 0.08571429 0.1 0.11428571 0.12857143 0.14285714 0.15714286 0.17142857 0.18571429 0.2 0.21428571 0.22857143 0.24285714 0.25714286 0.27142857 0.28571429 0.3 0.31428571 0.32857143 0.34285714 0.35714286 0.37142857 0.38571429 0.4 0.41428571 0.42857143 0.44285714 0.45714286 0.47142857 0.48571429 0.5 0.51428571 0.52857143 0.54285714 0.55714286 0.57142857 0.58571429 0.6 0.61428571 0.62857143 0.64285714 0.65714286 0.67142857 0.68571429 0.7 0.71428571 0.72857143 0.74285714 0.75714286 0.77142857 0.78571429 0.8 0.81428571 0.82857143 0.84285714 0.85714286 0.87142857 0.88571429 0.9 0.91428571 0.92857143 0.94285714 0.95714286 0.97142857 0.98571429 1 1 1 1 1 1
  arc A26 (4.321, 29.0182) -> (3.3214, 29.4323) centre (0, 20) ccw
  spline S13 degree 5 poles (3.3214, 29.4323) (3.3135, 29.4278) (3.2977, 29.4189) (3.2741, 29.4055) (3.2427, 29.3874) (3.2038, 29.3647) (3.1652, 29.3417) (3.1267, 29.3185) (3.0886, 29.295) (3.0507, 29.2714) (3.0131, 29.2476) (2.9757, 29.2235) (2.9386, 29.1992) (2.9018, 29.1748) (2.8652, 29.1501) (2.829, 29.1252) (2.793, 29.1001) (2.7573, 29.0748) (2.7218, 29.0493) (2.6867, 29.0236) (2.6518, 28.9977) (2.6173, 28.9716) (2.583, 28.9453) (2.549, 28.9187) (2.5153, 28.892) (2.482, 28.8651) (2.4489, 28.8381) (2.4162, 28.8108) (2.3837, 28.7833) (2.3516, 28.7556) (2.3198, 28.7278) (2.2883, 28.6997) (2.2572, 28.6715) (2.2264, 28.643) (2.1959, 28.6144) (2.1657, 28.5856) (2.1359, 28.5567) (2.1065, 28.5275) (2.0774, 28.4981) (2.0486, 28.4686) (2.0202, 28.4389) (1.9922, 28.409) (1.9646, 28.379) (1.9373, 28.3487) (1.9104, 28.3183) (1.8839, 28.2877) (1.8578, 28.2569) (1.8321, 28.226) (1.8067, 28.1948) (1.7818, 28.1636) (1.7573, 28.1321) (1.7332, 28.1005) (1.7096, 28.0686) (1.6865, 28.0366) (1.6639, 28.0045) (1.6417, 27.9721) (1.6199, 27.9396) (1.5985, 27.907) (1.5776, 27.8742) (1.5572, 27.8412) (1.5374, 27.808) (1.5182, 27.7746) (1.4998, 27.741) (1.4822, 27.7072) (1.4652, 27.6732) (1.4487, 27.639) (1.4326, 27.6047) (1.4169, 27.5704) (1.4017, 27.5359) (1.3875, 27.5013) (1.3747, 27.4662) (1.3661, 27.4377) (1.3609, 27.416) (1.3579, 27.4015) (1.3565, 27.3941) knots -1 -1 -1 -1 -1 -1 -0.98571429 -0.97142857 -0.95714286 -0.94285714 -0.92857143 -0.91428571 -0.9 -0.88571429 -0.87142857 -0.85714286 -0.84285714 -0.82857143 -0.81428571 -0.8 -0.78571429 -0.77142857 -0.75714286 -0.74285714 -0.72857143 -0.71428571 -0.7 -0.68571429 -0.67142857 -0.65714286 -0.64285714 -0.62857143 -0.61428571 -0.6 -0.58571429 -0.57142857 -0.55714286 -0.54285714 -0.52857143 -0.51428571 -0.5 -0.48571429 -0.47142857 -0.45714286 -0.44285714 -0.42857143 -0.41428571 -0.4 -0.38571429 -0.37142857 -0.35714286 -0.34285714 -0.32857143 -0.31428571 -0.3 -0.28571429 -0.27142857 -0.25714286 -0.24285714 -0.22857143 -0.21428571 -0.2 -0.18571429 -0.17142857 -0.15714286 -0.14285714 -0.12857143 -0.11428571 -0.1 -0.08571429 -0.07142857 -0.05714286 -0.04285714 -0.02857143 -0.01428571 0 0 0 0 0 0
  line L13 (1.3565, 27.3941) -> (1.0862, 25.9292)
  arc A27 (0.5454, 25.5223) -> (1.0862, 25.9292) centre (0.5945, 26.0199) ccw
  arc A28 (0.5454, 25.5223) -> (-0.5454, 25.5223) centre (0, 20) ccw
  arc A29 (-1.0862, 25.9292) -> (-0.5454, 25.5223) centre (-0.5945, 26.0199) ccw
  line L14 (-1.0862, 25.9292) -> (-1.3565, 27.3941)
  spline S14 degree 5 poles (-1.3565, 27.3941) (-1.3579, 27.4015) (-1.3609, 27.416) (-1.3661, 27.4377) (-1.3747, 27.4662) (-1.3875, 27.5013) (-1.4017, 27.5359) (-1.4169, 27.5704) (-1.4326, 27.6047) (-1.4487, 27.639) (-1.4652, 27.6732) (-1.4822, 27.7072) (-1.4998, 27.741) (-1.5182, 27.7746) (-1.5374, 27.808) (-1.5572, 27.8412) (-1.5776, 27.8742) (-1.5985, 27.907) (-1.6199, 27.9396) (-1.6417, 27.9721) (-1.6639, 28.0045) (-1.6865, 28.0366) (-1.7096, 28.0686) (-1.7332, 28.1005) (-1.7573, 28.1321) (-1.7818, 28.1636) (-1.8067, 28.1948) (-1.8321, 28.226) (-1.8578, 28.2569) (-1.8839, 28.2877) (-1.9104, 28.3183) (-1.9373, 28.3487) (-1.9646, 28.379) (-1.9922, 28.409) (-2.0202, 28.4389) (-2.0486, 28.4686) (-2.0774, 28.4981) (-2.1065, 28.5275) (-2.1359, 28.5567) (-2.1657, 28.5856) (-2.1959, 28.6144) (-2.2264, 28.643) (-2.2572, 28.6715) (-2.2883, 28.6997) (-2.3198, 28.7278) (-2.3516, 28.7556) (-2.3837, 28.7833) (-2.4162, 28.8108) (-2.4489, 28.8381) (-2.482, 28.8651) (-2.5153, 28.892) (-2.549, 28.9187) (-2.583, 28.9453) (-2.6173, 28.9716) (-2.6518, 28.9977) (-2.6867, 29.0236) (-2.7218, 29.0493) (-2.7573, 29.0748) (-2.793, 29.1001) (-2.829, 29.1252) (-2.8652, 29.1501) (-2.9018, 29.1748) (-2.9386, 29.1992) (-2.9757, 29.2235) (-3.0131, 29.2476) (-3.0507, 29.2714) (-3.0886, 29.295) (-3.1267, 29.3185) (-3.1652, 29.3417) (-3.2038, 29.3647) (-3.2427, 29.3874) (-3.2741, 29.4055) (-3.2977, 29.4189) (-3.3135, 29.4278) (-3.3214, 29.4323) knots 0 0 0 0 0 0 0.01428571 0.02857143 0.04285714 0.05714286 0.07142857 0.08571429 0.1 0.11428571 0.12857143 0.14285714 0.15714286 0.17142857 0.18571429 0.2 0.21428571 0.22857143 0.24285714 0.25714286 0.27142857 0.28571429 0.3 0.31428571 0.32857143 0.34285714 0.35714286 0.37142857 0.38571429 0.4 0.41428571 0.42857143 0.44285714 0.45714286 0.47142857 0.48571429 0.5 0.51428571 0.52857143 0.54285714 0.55714286 0.57142857 0.58571429 0.6 0.61428571 0.62857143 0.64285714 0.65714286 0.67142857 0.68571429 0.7 0.71428571 0.72857143 0.74285714 0.75714286 0.77142857 0.78571429 0.8 0.81428571 0.82857143 0.84285714 0.85714286 0.87142857 0.88571429 0.9 0.91428571 0.92857143 0.94285714 0.95714286 0.97142857 0.98571429 1 1 1 1 1 1
  arc A30 (-3.3214, 29.4323) -> (-4.321, 29.0182) centre (0, 20) ccw
  spline S15 degree 5 poles (-4.321, 29.0182) (-4.3235, 29.0095) (-4.3284, 28.992) (-4.3356, 28.9658) (-4.345, 28.9309) (-4.3564, 28.8873) (-4.3675, 28.8437) (-4.3782, 28.8001) (-4.3886, 28.7566) (-4.3987, 28.7131) (-4.4084, 28.6696) (-4.4179, 28.6261) (-4.4269, 28.5828) (-4.4357, 28.5394) (-4.444, 28.4961) (-4.4521, 28.4529) (-4.4598, 28.4097) (-4.4672, 28.3665) (-4.4742, 28.3234) (-4.4809, 28.2804) (-4.4872, 28.2374) (-4.4932, 28.1945) (-4.4988, 28.1517) (-4.5041, 28.1089) (-4.509, 28.0662) (-4.5136, 28.0236) (-4.5178, 27.9811) (-4.5217, 27.9386) (-4.5252, 27.8963) (-4.5283, 27.854) (-4.5311, 27.8118) (-4.5335, 27.7697) (-4.5356, 27.7277) (-4.5373, 27.6858) (-4.5386, 27.6441) (-4.5395, 27.6024) (-4.5401, 27.5608) (-4.5403, 27.5194) (-4.5402, 27.478) (-4.5396, 27.4368) (-4.5387, 27.3957) (-4.5374, 27.3548) (-4.5357, 27.314) (-4.5336, 27.2733) (-4.5311, 27.2328) (-4.5282, 27.1924) (-4.5249, 27.1522) (-4.5212, 27.1121) (-4.5171, 27.0722) (-4.5126, 27.0324) (-4.5077, 26.9928) (-4.5023, 26.9535) (-4.4965, 26.9143) (-4.4902, 26.8753) (-4.4835, 26.8365) (-4.4763, 26.798) (-4.4687, 26.7596) (-4.4607, 26.7214) (-4.4523, 26.6834) (-4.4434, 26.6457) (-4.434, 26.6082) (-4.424, 26.5711) (-4.4132, 26.5343) (-4.4018, 26.4979) (-4.3897, 26.4618) (-4.3772, 26.426) (-4.3643, 26.3904) (-4.3512, 26.355) (-4.3375, 26.3199) (-4.3231, 26.2853) (-4.3073, 26.2514) (-4.2932, 26.2253) (-4.2817, 26.2062) (-4.2734, 26.1938) (-4.2692, 26.1877) knots -1 -1 -1 -1 -1 -1 -0.98571429 -0.97142857 -0.95714286 -0.94285714 -0.92857143 -0.91428571 -0.9 -0.88571429 -0.87142857 -0.85714286 -0.84285714 -0.82857143 -0.81428571 -0.8 -0.78571429 -0.77142857 -0.75714286 -0.74285714 -0.72857143 -0.71428571 -0.7 -0.68571429 -0.67142857 -0.65714286 -0.64285714 -0.62857143 -0.61428571 -0.6 -0.58571429 -0.57142857 -0.55714286 -0.54285714 -0.52857143 -0.51428571 -0.5 -0.48571429 -0.47142857 -0.45714286 -0.44285714 -0.42857143 -0.41428571 -0.4 -0.38571429 -0.37142857 -0.35714286 -0.34285714 -0.32857143 -0.31428571 -0.3 -0.28571429 -0.27142857 -0.25714286 -0.24285714 -0.22857143 -0.21428571 -0.2 -0.18571429 -0.17142857 -0.15714286 -0.14285714 -0.12857143 -0.11428571 -0.1 -0.08571429 -0.07142857 -0.05714286 -0.04285714 -0.02857143 -0.01428571 0 0 0 0 0 0
  line L15 (-4.2692, 26.1877) -> (-3.4245, 24.9606)
  arc A31 (-3.5192, 24.2905) -> (-3.4245, 24.9606) centre (-3.8363, 24.6771) ccw
  arc A32 (-2, 17.9) -> (2, 17.9) centre (0, 20) ccw
  line L16 (-2, 17.9) -> (-2, 22.1)
  arc A33 (2, 22.1) -> (-2, 22.1) centre (0, 20) ccw
  line L17 (2, 22.1) -> (2, 17.9)
  circle A34 centre (0, 20) radius 2.9
  dimension "d63" = 5.8
  constraint concentric A0 A34
  measures "d63" diameter of A34
extrude "Extrude4" cut sketch "Sketch8" against normal blind 4 contours A32 L16 A33 L17 A34 | L16 A34 | L17 A34 sketch seen with x (0.92388, 0.382683, 0) y (-0.382683, 0.92388, 0) z (0, 0, 1) at (-7.6537, 18.4776, 0) bodies 2 in component "Spur Gear (8 teeth)"
move_face "OffsetFaces1" offset 1 1 faces at (4.4729, -0.5714, 4) on bodies 1 in component "Spur Gear (12 teeth)"
move_face "OffsetFaces1'" offset 1 1 faces at (0.0452, -4.615, 4) on bodies 2 in component "Spur Gear (8 teeth)"
component "Spur Gear (12 teeth)" placed x (1, 0, 0) y (0, 1, 0) z (0, 0, 1) at (0, 0, 0)
component "Spur Gear (8 teeth)" placed x (0.92388, -0.382683, 0) y (0.382683, 0.92388, 0) z (0, 0, 1) at (0, -20, 0)
equation "distanceOne = 4.00 mm"
equation "taperAngle1 = 0.0 deg"
equation "Radius = 0.50 mm"
equation "countU = 12"

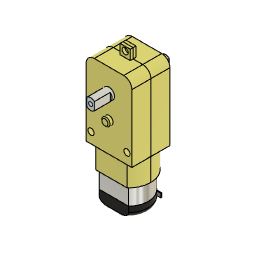
design "DC 3777"
Autodesk Fusion 360 part; units mm, degrees
sketch "main" plane through (0, 0, 0) normal (0, 1, 0) x (1, 0, 0)
  circle A0 centre (0, 0) radius 2.7
  line L0 (-11.2, -11.2) -> (11.2, -11.2)
  line L1 (11.2, -11.2) -> (11.2, 51)
  line L2 (11.2, 51) -> (-11.2, 51)
  line L3 (-11.2, 51) -> (-11.2, -11.2)
  line L4 (0, -11.2) -> (0, 51) construction
  line L5 (-2.5, -16) -> (2.5, -16)
  line L6 (2.5, -16) -> (2.5, -11.2)
  line L7 (2.5, -11.2) -> (-2.5, -11.2)
  line L8 (-2.5, -11.2) -> (-2.5, -16)
  circle A1 centre (0, -14) radius 1.5
  line L9 (-11.2, 25.8) -> (11.2, 25.8)
  line L10 (-1.85, 2.7) -> (1.85, 2.7)
  line L11 (1.85, 2.7) -> (1.85, -2.7)
  line L12 (1.85, -2.7) -> (-1.85, -2.7)
  line L13 (-1.85, -2.7) -> (-1.85, 2.7)
  line L14 (-1.85, 2.7) -> (1.85, -2.7) construction
  line L15 (1.85, 2.7) -> (-1.85, -2.7) construction
  circle A2 centre (8.8, 20.6) radius 1.5
  circle A3 centre (-8.8, 20.6) radius 1.5
  line L16 (8.8, 20.6) -> (-8.8, 20.6) construction
  circle A4 centre (0, 0) radius 0.975
  line L17
  dimension "d1" = 5.4
  dimension "d2" = 22.4
  dimension "d3" = 62.2
  dimension "d4" = 11.2
  dimension "d5" = 5
  dimension "d7" = 3
  dimension "d8" = 2
  dimension "d10" = 3.7
  dimension "d11" = 5.4
  dimension "d21" = 3
  dimension "d22" = 8.8
  dimension "d23" = 3
  dimension "d24" = 8.8
  dimension "d25" = 31.8
  dimension "d52" = 37
  dimension "d61" = 1.95
  dimension "d62" = 4.8
  constraint coincident A0.centre A4.centre
  constraint horizontal L0
  constraint vertical L1
  constraint horizontal L2
  constraint vertical L3
  constraint midpoint L0 L4.start
  constraint midpoint L2 L4.end
  constraint coincident A0.centre L4
  constraint horizontal L5
  constraint vertical L6
  constraint horizontal L7
  constraint vertical L8
  constraint midpoint L0 L7
  constraint coincident L3 L9.start
  constraint coincident L1 L9.end
  constraint perpendicular L1 L9
  constraint perpendicular L10 L11
  constraint parallel L10 L12
  constraint parallel L11 L13
  constraint horizontal L10
  constraint coincident L14 A0.centre
  constraint coincident L15 A0.centre
  constraint coincident A2.centre L16.start
  constraint coincident A3.centre L16.end
  constraint horizontal L16
  measures "d1" diameter of A0
  measures "d2" distance of L0.start L0.end
  measures "d3" distance of L0.end L1.end
  measures "d4" distance of A0.centre L0
  measures "d5" distance of L5.start L5.end
  measures "d7" diameter of A1
  measures "d8" distance of L5 A1.centre
  measures "d10" distance of L11.end L12.end
  measures "d11" distance of L10.end L11.end
  measures "d21" diameter of A2
  measures "d22" distance of L4 A2.centre
  measures "d23" diameter of A3
  measures "d24" distance of L4 A3.centre
  measures "d25" distance of L0 A2.centre
  measures "d52" distance of L0 L9
  measures "d61" diameter of A4
  measures "d62" distance of L5.end L6.end
extrude "Extrude1" add sketch "main" along normal mid plane 18.6 contours A0 L10 L11 | A0 L11 L12 | A0 L10 L13 | A0 L12 L13 | L0 L1 L3 L7 L9 makes body 1
extrude "Extrude2" add sketch "main" along normal mid plane 2.8 contours L0 L5 L6 L7 L8 bodies 1
extrude "Extrude3" add sketch "main" along normal mid plane 21 separate body contours A0 L11 | A0 L11 L13 | A0 L13 | A4 makes body 2
extrude "Extrude4" add sketch "main" along normal mid plane 36.6 contours A0 L11 L13 bodies 2
fillet "Fillet1" radius 4 2 edges at (11.2, 0, 11.2) (-11.2, 0, 11.2) on bodies 1
sketch "bottom" plane through (0, 0, -25.8) normal (0, 0, -1) x (1, 0, 0)
  line L0 (-11.2, 9.3) -> (-11.2, -9.3)
  line L1 (-11.2, -9.3) -> (11.2, -9.3)
  line L2 (11.2, -9.3) -> (11.2, 9.3)
  line L3 (11.2, 9.3) -> (-11.2, 9.3)
  circle A0 centre (0, 0) radius 11.15
  line L4 (-11.2, 8.1) -> (11.2, 8.1)
  dimension "d26" = 22.3
  dimension "d29" = 1.2
  constraint coincident A0.centre origin
  constraint coincident L0 L4.start
  constraint coincident L2 L4.end
  constraint horizontal L4
  measures "d26" diameter of A0
  measures "d29" distance of L3 L4
extrude "Extrude5" add sketch "bottom" along normal blind 11 contours L1 A0 L4 bodies 1
sketch "more" plane through (0, 0, -36.8) normal (0, 0, -1) x (1, 0, 0)
  arc A0 (-7.6624, 8.1) -> (-6.1508, -9.3) centre (0, 0) ccw
  line L0 (-6.1508, -9.3) -> (6.1508, -9.3)
  arc A1 (6.1508, -9.3) -> (7.6624, 8.1) centre (0, 0) ccw
  line L1 (7.6624, 8.1) -> (-7.6624, 8.1)
  circle A2 centre (0, 0) radius 4.95
  arc A3 (-7.1689, 6.9) -> (-5.7786, -8.1) centre (0, 0) ccw
  line L2 (-5.7786, -8.1) -> (5.7786, -8.1)
  arc A4 (5.7786, -8.1) -> (7.1689, 6.9) centre (0, 0) ccw
  line L3 (7.1689, 6.9) -> (-7.1689, 6.9)
  line L4 (-5, 3.6) -> (5, 3.6)
  circle A5 centre (0, 0) radius 1
  dimension "d30" = 9.9
  dimension "d31" = 1.2
  dimension "d37" = 3.6
  dimension "d41" = 2
  constraint coincident A0.centre A1.centre
  constraint parallel L3 L4
  measures "d30" diameter of A2
  measures "d37" distance of A0.centre L4
  measures "d41" diameter of A5
extrude "Extrude6" add sketch "more" along normal blind 8.6 separate body contours A2 L4 | A2 L4 | A3 L2 A4 L3 | A5 makes body 3
extrude "Extrude7" add sketch "more" along normal blind 5.2 from surface at 8.6 separate body contours A2 L4 | A2 L4 | A3 L2 A4 L3 | A5 makes body 4
extrude "Extrude8" add sketch "more" along normal blind 2 from surface at 13.8 contours A2 L4 | A5 picked at (-0.0249, 2.7324) bodies 4
extrude "Extrude9" add sketch "more" along normal blind 2 from surface at 15.8 separate body contours A5 makes body 5
fillet "Fillet2" radius 1 1 edges at (-0.9323, 0.3616, -54.6) on bodies 5
sketch "nubber" plane through (0, -9.3, 0) normal (0, -1, 0) x (1, 0, 0)
  circle A0 centre (-8.8, -20.6) radius 1.5
  circle A1 centre (8.8, -20.6) radius 1.5
  arc A2 (-7.2, 11.2) -> (-11.2, 7.2) centre (-7.2, 7.2) ccw
  line L0 (-11.2, 7.2) -> (-11.2, -25.8)
  line L1 (-11.2, -25.8) -> (11.2, -25.8)
  line L2 (11.2, -25.8) -> (11.2, 7.2)
  arc A3 (11.2, 7.2) -> (7.2, 11.2) centre (7.2, 7.2) ccw
  line L3 (7.2, 11.2) -> (-7.2, 11.2)
  circle A4 centre (0, -11.25) radius 2
  circle A5 centre (0, 0) radius 2.7
  line L4
  dimension "d46" = 4
  dimension "d47" = 11.25
  measures "d46" diameter of A4
  measures "d47" distance of A5.centre A4.centre
extrude "Extrude10" add sketch "nubber" along normal blind 2 contours A4 bodies 1
fillet "Fillet3" radius 0.5 1 edges at (-1.8647, -11.3, -11.9732) on bodies 1
fillet "Fillet4" radius 2.5 2 edges at (-9.9075, 0.9183, -50.6) (9.9075, 0.9183, -50.6) on bodies 4
split "Split1" by plane through (0, 0, 0) normal (0, 1, 0) bodies 1 makes body 6 at (0.0673, 9.3, -13.9506)
sketch "Sketch5" plane through (0, 8.1, 0) normal (0, 1, 0) x (-1, 0, 0)
  spline S0 degree 3 poles (5.7786, -48.1) (5.7786, -48.2998) (5.7259, -48.5338) (5.5453, -48.9398) (5.3678, -49.1736) (4.9234, -49.5927) (4.5434, -49.8136) (3.5837, -50.2134) (2.8684, -50.347) (1.4131, -50.4957) (0.6733, -50.514) (-0.6733, -50.514) (-1.4131, -50.4957) (-2.8684, -50.347) (-3.5837, -50.2134) (-4.5434, -49.8136) (-4.9234, -49.5927) (-5.3678, -49.1736) (-5.5453, -48.9398) (-5.7259, -48.5338) (-5.7786, -48.2998) (-5.7786, -48.1) knots 0.647214 0.647214 0.647214 0.647214 0.707165 0.707165 0.780538 0.780538 0.890431 0.890431 1.09243 1.09243 1.294429 1.294429 1.496428 1.496428 1.698427 1.698427 1.80832 1.80832 1.881693 1.881693 1.941643 1.941643 1.941643 1.941643
  line L0 (5.7786, -48.1) -> (5.7786, -45.4)
  line L1 (5.7786, -45.4) -> (-5.7786, -45.4)
  line L2 (-5.7786, -45.4) -> (-5.7786, -48.1)
  line L3 (-2, -47) -> (-8, -47)
  line L4 (-8, -47) -> (-8, -49)
  line L5 (-8, -49) -> (-2, -49)
  line L6 (-2, -49) -> (-2, -47)
  line L7 (2, -47) -> (8, -47)
  line L8 (8, -47) -> (8, -49)
  line L9 (8, -49) -> (2, -49)
  line L10 (2, -49) -> (2, -47)
  line L11
  dimension "d53" = 6
  dimension "d54" = 2
  dimension "d55" = 2
  dimension "d56" = 6
  dimension "d57" = 2
  dimension "d58" = 4
  constraint horizontal L3
  constraint vertical L4
  constraint horizontal L5
  constraint vertical L6
  constraint horizontal L7
  constraint vertical L8
  constraint horizontal L9
  constraint vertical L10
  measures "d53" distance of L3.start L3.end
  measures "d54" distance of L3.start L5.end
  measures "d55" distance of origin L6
  measures "d56" distance of L7.start L7.end
  measures "d57" distance of L7.start L9.end
  measures "d58" distance of L6 L10
extrude "Extrude11" add sketch "Sketch5" along normal blind 0.4 separate body contours S0 L0 L7 L8 L9 | S0 L0 L7 L9 L10 | S0 L2 L3 L4 L5 | S0 L2 L3 L5 L6 makes body 7 at (-4, 8.1, -47.6667) makes body 8 at (4, 8.1, -48.3333)
sketch "Sketch6" plane through (0, -18.3, 0) normal (0, -1, 0) x (1, 0, 0)
  circle A0 centre (0, 0) radius 0.975
  arc A1 (-1.85, -1.9666) -> (1.85, -1.9666) centre (0, 0) ccw
  line L0 (1.85, -1.9666) -> (1.85, 1.9666)
  arc A2 (1.85, 1.9666) -> (-1.85, 1.9666) centre (0, 0) ccw
  line L1
equation "d22 = ( 17.6 / 2 ) * 1 mm"
equation "d24 = ( 17.6 / 2 ) * 1 mm"
named bodies: "body A", "shaft", "metal bit", "cap", "pin thingy", "body B", "anode", "cathy"

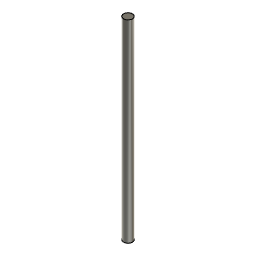
design "Rear axle"
Autodesk Fusion 360 part; units mm, degrees
sketch "Sketch1" plane through (0, 0, 0) normal (0, 0, 1) x (1, 0, 0)
  circle A0 centre (0, 0) radius 2.75
  dimension "d1" = 5.5
  constraint coincident A0.centre origin
  measures "d1" diameter of A0
extrude "Extrude1" add sketch "Sketch1" along normal blind 120
